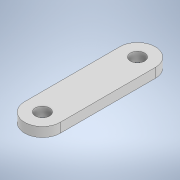
# Autodesk Inventor part: Cable_Guide_Holder_Block
Saved by Autodesk Inventor 2021 (Build 250183000, 183)
## iProperties
Created: 2022-01-10
Part Number: Cable_Guide_Holder_Block
Material: Generic
Document SubType Name: Modeling
Designer: Jorian Brusind
Density: 1 g/cm^3
Appearance: Default
Author: Jorian Brusind
Autodesk Inventor part; units mm, degrees
ref_plane "YZ Plane" through (0, 0, 0) normal (1, 0, 0) x (0, 1, 0)
ref_plane "XZ Plane" through (0, 0, 0) normal (0, 1, 0) x (-1, 0, 0)
ref_plane "XY Plane" through (0, 0, 0) normal (0, 0, 1) x (1, 0, 0)
sketch "Sketch1" plane through (0, 0, 0) normal (0, 1, 0) x (-1, 0, 0)
  line L0 (0, 20) -> (0, -20) construction
  line L1 (-7.5, 20) -> (-7.5, -20)
  line L2 (7.5, -20) -> (7.5, 20)
  arc A0 (7.5, 20) -> (-7.5, 20) centre (0, 20) ccw
  arc A1 (-7.5, -20) -> (7.5, -20) centre (0, -20) ccw
  line L3 (0, 0) -> (40, 0) construction
  circle A2 centre (0, -20) radius 3
  circle A3 centre (0, 20) radius 3
  dimension "d1" = 20
  dimension "d2" = 90
  dimension "d3" = 15
  dimension "d4" = 6
  dimension "d5" = 6
  constraints: 10 end point, 4 centre point, 4 point on circle, 4 tangent, 3 coincident, 1 horizontal, 1 midpoint, 1 parallel, 1 perpendicular, 1 vertical
  measures "d1" distance of L3.start L0.end
  measures "d2" angle of L0 L3
  measures "d3" diameter of A1
  measures "d4" diameter of A2
  measures "d5" diameter of A3
extrude "Extrusion1" add sketch "Sketch1" along normal blind 4
body "Solid1"
